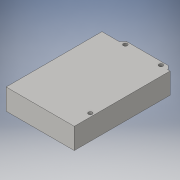
# Autodesk Inventor part: Arduino board with Sheild
Saved by Autodesk Inventor 2016 (Build 200138000, 138)
## iProperties
Created: 2017-10-12
Part Number: Arduino board with Sheild
Material: Generic
Document SubType Name: Modeling
Designer: Student
Density: 1 g/cm^3
Appearance: Default
Author: Student
Autodesk Inventor part; units mm, degrees
ref_plane "YZ Plane" through (0, 0, 0) normal (1, 0, 0) x (0, 1, 0)
ref_plane "XZ Plane" through (0, 0, 0) normal (0, 1, 0) x (-1, 0, 0)
ref_plane "XY Plane" through (0, 0, 0) normal (0, 0, 1) x (1, 0, 0)
sketch "Sketch1" plane through (0, 0, 0) normal (0, 1, 0) x (-1, 0, 0)
  line L0 (9.5985, 62.4723) -> (-43.8177, 62.4723)
  line L1 (-43.8177, 62.4723) -> (-43.8177, -12.6609)
  line L2 (-43.8177, -12.6609) -> (9.5985, -12.6609)
  line L3 (9.5985, -12.6609) -> (9.5985, 62.4723)
  line L4 (-41.7857, -12.6609) -> (-4.3715, -12.6609)
  line L5 (-4.3715, -12.6609) -> (-4.3715, -15.6073)
  line L6 (-4.3715, -15.6073) -> (-41.7857, -15.6073)
  line L7 (-41.7857, -15.6073) -> (-41.7857, -12.6609)
  point P0 (0, 0)
  dimension "d0" = 75.1332
  dimension "d1" = 53.4162
  dimension "d2" = 37.4142
  dimension "d3" = 2.032
  dimension "d4" = 2.9464
  constraints: 16 end point, 4 parallel, 2 horizontal, 2 perpendicular, 1 point on line
  measures "d0" distance of L2.end L0.start
  measures "d1" distance of L1.end L2.end
  measures "d2" distance of L5.end L6.end
  measures "d3" distance between parallel lines of L7 L1
  measures "d4" distance of L4.end L5.end
extrude "Extrusion1" add sketch "Sketch1" along normal blind 16.4338
chamfer "Chamfer1" distance 2.54 angle 45 2 edges at (41.7857, 8.2169, -15.6073) (4.3715, 8.2169, -15.6073)
sketch "Sketch2" plane through (0, 16.4338, 0) normal (0, 1, 0) x (1, 0, 0)
  circle A0 centre (8.3974, 12.9784) radius 1.5367
  circle A1 centre (36.2866, 12.9784) radius 1.5367
  line L0 (39.2457, 15.6073) -> (6.9115, 15.6073) projected
  line L1 (43.8177, -62.4723) -> (43.8177, 12.6609) projected
  circle A2 centre (41.1761, -47.2577) radius 1.5367
  line L2 (-9.5985, -62.4723) -> (43.8177, -62.4723) projected
  point P0 (0, 0)
  dimension "d10" = 3.0734
  dimension "d11" = 2.6289
  dimension "d12" = 3.0734
  dimension "d13" = 2.6289
  dimension "d14" = 7.5311
  dimension "d15" = 27.8892
  dimension "d16" = 15.2146
  dimension "d17" = 2.6416
  dimension "d18" = 3.0734
  dimension "d21" = 60.2361
  dimension "d22" = 4.8895
  constraints: 3 centre point
  measures "d10" diameter of A0
  measures "d11" distance from line of L0 A0.centre
  measures "d12" diameter of A1
  measures "d13" distance from line of L0 A1.centre
  measures "d14" distance from line of L1 A1.centre
  measures "d15" distance of A1.centre A0.centre
  measures "d16" distance from line of A2.centre L2
  measures "d17" distance from line of L1 A2.centre
  measures "d18" diameter of A2
  measures "d21" vertical distance of A2.centre A1.centre
  measures "d22" horizontal distance of A1.centre A2.centre
extrude "Extrusion2" cut sketch "Sketch2" against normal blind 16.4338
equation "\"d13\" = d11"
equation "\"d18\" = d12"
body "Solid1"
